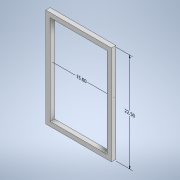
# Autodesk Inventor part: primative4thStageForShortRobot
Saved by Autodesk Inventor 2020.2 (Build 242310000, 310)
## iProperties
Created: 2020-01-09
Part Number: primative4thStageForShortRobot
Material: Generic
Document SubType Name: Modeling
Designer: steele
Density: 1 g/cm^3
Appearance: Default
Author: steele
Autodesk Inventor part; units mm, degrees
ref_plane "YZ Plane" through (0, 0, 0) normal (1, 0, 0) x (0, 1, 0)
ref_plane "XZ Plane" through (0, 0, 0) normal (0, 1, 0) x (-1, 0, 0)
ref_plane "XY Plane" through (0, 0, 0) normal (0, 0, 1) x (1, 0, 0)
sketch "Sketch1" plane through (0, 0, 0) normal (0, 0, 1) x (1, 0, 0)
  line L0 (0, 0) -> (190.5, 0)
  line L1 (190.5, 0) -> (190.5, 571.5)
  line L2 (190.5, 571.5) -> (0, 571.5)
  line L3 (0, 0) -> (0, 571.5) construction
  line L4 (0, 0) -> (-190.5, 0)
  line L5 (-190.5, 0) -> (-190.5, 571.5)
  line L6 (-190.5, 571.5) -> (0, 571.5)
  line L7 (-165.1, 25.4) -> (165.1, 25.4)
  line L8 (165.1, 25.4) -> (165.1, 546.1)
  line L9 (165.1, 546.1) -> (-165.1, 546.1)
  line L10 (-165.1, 546.1) -> (-165.1, 25.4)
  dimension "d1" = 571.5
  dimension "d2" = 381
  dimension "d3" = 25.4
  dimension "d4" = 25.4
  dimension "d5" = 25.4
  dimension "d6" = 25.4
  constraints: 22 end point, 3 parallel, 2 horizontal, 2 perpendicular, 2 symmetric about line, 1 vertical
  measures "d1" distance of L1.end L0.end
  measures "d2" distance between parallel lines of L1 L5
  measures "d3" distance between parallel lines of L7 L0
  measures "d4" distance between parallel lines of L1 L8
  measures "d5" distance between parallel lines of L2 L9
  measures "d6" distance between parallel lines of L5 L10
extrude "Extrusion1" add sketch "Sketch1" along normal mid plane 25.4
body "Solid1"
